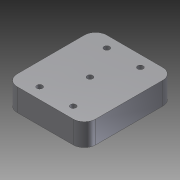
# Autodesk Inventor part: Fixed Extension
Saved by Autodesk Inventor 2012 (Build 160160000, 160)
## iProperties
Created: 2011-10-21
Part Number: Fixed Extension
Material: Default
Document SubType Name: Modeling
Designer: Robotics
Density: 1 g/cm^3
Author: Robotics
Autodesk Inventor part; units mm, degrees
ref_plane "YZ Plane" through (0, 0, 0) normal (1, 0, 0) x (0, 1, 0)
ref_plane "XZ Plane" through (0, 0, 0) normal (0, 1, 0) x (-1, 0, 0)
ref_plane "XY Plane" through (0, 0, 0) normal (0, 0, 1) x (1, 0, 0)
sketch "Sketch2" plane through (0, 0, 0) normal (0, 1, 0) x (-1, 0, 0)
  line L0 (-44.45, 50.8) -> (44.45, 50.8)
  line L1 (44.45, 50.8) -> (44.45, -50.8)
  line L2 (44.45, -50.8) -> (-44.45, -50.8)
  line L3 (-44.45, -50.8) -> (-44.45, 50.8)
  point P0 (0, 0)
  dimension "d0" = 44.45
  dimension "d1" = 44.45
  dimension "d2" = 50.8
  dimension "d3" = 50.8
  constraints: 8 end point, 2 parallel, 1 horizontal, 1 perpendicular
  measures "d0" distance from line of L1 point (0, 0)
  measures "d1" distance from line of L3 point (0, 0)
  measures "d2" distance from line of L2 point (0, 0)
  measures "d3" distance from line of L0 point (0, 0)
extrude "Extrusion1" add sketch "Sketch2" along normal blind 25.4
fillet "Fillet1" radius 12.7 4 edges at (44.45, 12.7, 50.8) (-44.45, 12.7, 50.8) (44.45, 12.7, -50.8) (-44.45, 12.7, -50.8)
sketch "Sketch3" plane through (0, 25.4, 0) normal (0, 1, 0) x (1, 0, 0)
  line L0 (-44.45, -38.1) -> (-44.45, 38.1) projected
  line L1 (31.75, -50.8) -> (-31.75, -50.8) projected
  line L2 (44.45, 38.1) -> (44.45, -38.1) projected
  line L3 (-31.75, 50.8) -> (31.75, 50.8) projected
  point P0 (0, 0)
  point P1 (-19.05, 38.1)
  point P2 (19.05, 38.1)
  point P3 (19.05, -38.1)
  point P4 (-19.05, -38.1)
  point P5 (0, 0)
  dimension "d7" = 25.4
  dimension "d8" = 25.4
  dimension "d9" = 12.7
  dimension "d10" = 12.7
  constraints: 2 horizontal alignment, 2 vertical alignment, 1 coincident
  measures "d7" distance from line of L0 point (-19.05, 38.1)
  measures "d8" distance from line of L2 point (19.05, 38.1)
  measures "d9" distance from line of L3 point (-19.05, 38.1)
  measures "d10" distance from line of L1 point (-19.05, -38.1)
hole "Hole1" at (-19.05, 25.4, -38.1) at (19.05, 25.4, -38.1) at (19.05, 25.4, 38.1) at (-19.05, 25.4, 38.1) at (0, 25.4, 0) direction (0, -1, 0) diameter 6.35 end through all
equation "\"d1\" = d0"
equation "\"d3\" = d2"
equation "\"d8\" = d7"
body "Solid1"
